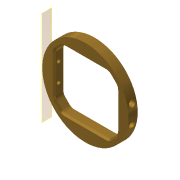
# Autodesk Inventor part: Radial Bushing
Saved by Autodesk Inventor 2014 SP1 (Build 180222100, 222)
## iProperties
Created: 2014-04-22
Part Number: Radial Bushing
Material: Generic
Document SubType Name: Modeling
Designer: Rauhul Varma
Density: 1 g/cm^3
Appearance: Brass - Satin
Author: Rauhul Varma
Autodesk Inventor part; units mm, degrees
ref_plane "XZ Plane" through (0, 0, 0) normal (0, 1, 0) x (-1, 0, 0)
ref_plane "XY Plane" through (0, 0, 0) normal (0, 0, 1) x (1, 0, 0)
sketch "Sketch1" plane through (0, 0, 0) normal (0, 0, 1) x (1, 0, 0)
  circle A0 centre (0, 0) radius 44.45
  line L0 (-32.2263, -21.7487) -> (32.2263, -21.7487)
  line L1 (32.2263, -21.7487) -> (32.2263, 21.7487)
  line L2 (32.2263, 21.7487) -> (-32.2263, 21.7487)
  line L3 (-32.2263, 21.7487) -> (-32.2263, -21.7487)
  line L4 (-32.2263, -21.7487) -> (32.2263, 21.7487) construction
  line L5 (32.2263, -21.7487) -> (-32.2263, 21.7487) construction
  line L6 (-23.8125, -30.1625) -> (23.8125, -30.1625)
  line L7 (23.8125, -30.1625) -> (23.8125, 30.1625)
  line L8 (23.8125, 30.1625) -> (-23.8125, 30.1625)
  line L9 (-23.8125, 30.1625) -> (-23.8125, -30.1625)
  line L10 (-23.8125, -30.1625) -> (23.8125, 30.1625) construction
  line L11 (23.8125, -30.1625) -> (-23.8125, 30.1625) construction
  line L12 (-32.2263, 21.7487) -> (-23.8125, 30.1625)
  line L13 (-32.2263, -21.7487) -> (-23.8125, -30.1625)
  line L14 (23.8125, -30.1625) -> (32.2263, -21.7487)
  line L15 (32.2263, 21.7487) -> (23.8125, 30.1625)
  dimension "d0" = 88.9
  dimension "d2" = 64.4525
  dimension "d5" = 47.625
  dimension "d6" = 60.325
  dimension "d18" = 45
  constraints: 32 end point, 5 parallel, 4 midpoint, 2 horizontal, 2 perpendicular, 1 centre point, 1 coincident
  measures "d0" diameter of A0
  measures "d2" distance of L1.end L2.end
  measures "d5" distance of L8.end L7.end
  measures "d6" distance of L8.end L6.start
  measures "d18" angle of L12 L2
extrude "Extrusion1" add sketch "Sketch1" along normal blind 9.525
fillet "Fillet1" radius 6.096 8 edges at (23.8125, -30.1625, 4.7625) (32.2263, -21.7487, 4.7625) (23.8125, 30.1625, 4.7625) (32.2263, 21.7487, 4.7625) (-23.8125, 30.1625, 4.7625) (-32.2263, 21.7487, 4.7625) (-32.2263, -21.7487, 4.7625) (-23.8125, -30.1625, 4.7625)
ref_plane "Work Plane1" through (-44.45, 0, 0) normal (1, 0, 0) x (0, 1, 0)
sketch "Sketch2" plane through (-44.45, 0, 0) normal (1, 0, 0) x (0, 1, 0)
  line L0 (19.2237, 0) -> (-19.2237, 0) projected
  line L1 (-19.2237, 9.525) -> (19.2237, 9.525) projected
  line L2 (0, 9.525) -> (0, 0) construction
  line L3 (-20.6375, 4.7625) -> (20.6375, 4.7625) construction
  line L4 (-19.2237, 0) -> (-19.2237, 9.525) projected
  line L5 (19.2237, 9.525) -> (19.2237, 0) projected
  point P0 (-9.525, 4.7625)
  point P1 (9.525, 4.7625)
  dimension "d9" = 19.05
  dimension "d10" = 9.525
  constraints: 4 end point, 2 point on line, 1 midpoint, 1 perpendicular
  measures "d9" distance of point (-9.525, 4.763) point (9.525, 4.763)
  measures "d10" distance from line of L2 point (-9.525, 4.763)
hole "Hole1" at (-44.45, -9.525, 4.7625) at (-44.45, 9.525, 4.7625) direction (1, 0, 0) diameter 3.6576 end up to face face through (-32.2263, 6.4079, 6.35) facing (1, 0, 0) counterbore diameter 6.35 counterbore depth 5.715 clearance for "Socket Head Cap Screw" size "#6" standard "Ansi Unified Screw Threads"
mirror "Mirror1" about plane through (0, 0, 0) normal (1, 0, 0) of "Hole1"
chamfer "Chamfer1" distance 1.5875 angle 45 16 edges at (0, -30.1625, 9.525) (-23.6203, -29.6985, 9.525) (-28.0194, -25.9556, 9.525) (-31.7622, -21.5565, 9.525) (-32.2263, 0, 9.525) (-31.7622, 21.5565, 9.525) (-28.0194, 25.9556, 9.525) (-23.6203, 29.6985, 9.525) (0, 30.1625, 9.525) (23.6203, 29.6985, 9.525) (28.0194, 25.9556, 9.525) (31.7622, 21.5565, 9.525) (32.2263, 0, 9.525) (31.7622, -21.5565, 9.525) (28.0194, -25.9556, 9.525) (23.6203, -29.6985, 9.525)
equation "\"d10\" = 0.5 * d9"
body "Solid1"
